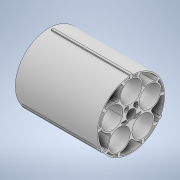
# Autodesk Inventor part: Engine
Saved by Autodesk Inventor 2020 (Build 240168000, 168)
## iProperties
Created: 2022-02-05
Part Number: Engine
Material: Generisch
Document SubType Name: Modeling
Designer: sp
Density: 1 g/cm^3
Appearance: Vorgabe
Author: sp
Autodesk Inventor part; units mm, degrees
ref_plane "YZ Plane" through (0, 0, 0) normal (1, 0, 0) x (0, 1, 0)
ref_plane "XZ Plane" through (0, 0, 0) normal (0, 1, 0) x (-1, 0, 0)
ref_plane "XY Plane" through (0, 0, 0) normal (0, 0, 1) x (1, 0, 0)
sketch "Skizze1" plane through (0, 0, 0) normal (1, 0, 0) x (0, 1, 0)
  circle A0 centre (0, 0) radius 30 construction
  circle A1 centre (17.5, 0) radius 9.5
  circle A2 centre (17.5, 0) radius 10.5
  circle A3 centre (5.4078, 16.6435) radius 9.5
  circle A4 centre (5.4078, 16.6435) radius 10.5
  circle A5 centre (-14.1578, 10.2862) radius 9.5
  circle A6 centre (-14.1578, 10.2862) radius 10.5
  circle A7 centre (-14.1578, -10.2862) radius 9.5
  circle A8 centre (-14.1578, -10.2862) radius 10.5
  circle A9 centre (5.4078, -16.6435) radius 9.5
  circle A10 centre (5.4078, -16.6435) radius 10.5
  circle A11 centre (0, 0) radius 4
  circle A12 centre (0, 0) radius 30
  circle A13 centre (0, 0) radius 29
  dimension "d0" = 60
  dimension "d1" = 17.5
  dimension "d2" = 19
  dimension "d3" = 21
  dimension "d6" = 360
  dimension "d8" = 8
  dimension "d12" = 58
  constraints: 14 centre point, 14 coincident, 1 concentric, 31 other
  measures "d0" diameter of A0
  measures "d1" distance of point (0, 0) point (17.5, 0)
  measures "d2" diameter of A1
  measures "d3" diameter of A2
  measures "d8" diameter of A11
  measures "d12" diameter of A13
extrude "Extrusion1" add sketch "Skizze1" against normal mid plane 70 contours A2 A10 A4 | A4 A2 | A2 A4 A6 | A10 A8 A2 | A2 A10 | A6 A8 A4 | A4 A6 | A10 A8 A6 | A8 A10 | A8 A6
fillet "Rundung1" radius 2 10 edges at (0, 13.1592, -9.5607) (0, -5.0264, -15.4696) (0, -16.2657, 0) (0, -5.0264, 15.4696) (0, 13.1592, 9.5607) (0, 9.7486, -7.0828) (0, 9.7486, 7.0828) (0, -3.7236, 11.4601) (0, -12.0499, 0) (0, -3.7236, -11.4601)
sketch "Skizze2" plane through (35, 0, 0) normal (1, 0, 0) x (0, 0, -1)
  circle A0 centre (0, 0) radius 30
  circle A1 centre (0, 0) radius 29
  dimension "d13" = 60
  dimension "d14" = 58
  constraints: 2 centre point, 2 coincident
  measures "d13" diameter of A0
  measures "d14" diameter of A1
extrude "Extrusion2" add sketch "Skizze2" against normal blind 70
sketch "Skizze3" plane through (0, 0, 0) normal (1, 0, 0) x (0, 1, 0)
  line L0 (35.299, 0) -> (22.394, 0) construction
  line L1 (46.9219, 0) -> (-63.2802, 0) construction
  arc A0 (17.2478, -10.497) -> (17.2478, 10.497) centre (17.5, 0) ccw projected
  line L2 (27.9523, 1) -> (30.9523, 1)
  line L3 (30.9523, 1) -> (30.9523, -1)
  line L4 (30.9523, -1) -> (27.9523, -1)
  line L5 (27.9523, -1) -> (27.9523, 1)
  point P0 (0, 0)
  point P1 (29.9278, 0)
  dimension "d17" = 2
  dimension "d18" = 3
  constraints: 12 end point, 3 horizontal, 3 point on line, 2 parallel, 1 perpendicular, 1 point on circle, 1 other
  measures "d17" distance between parallel lines of L4 L2
  measures "d18" distance between parallel lines of L5 L3
extrude "Extrusion3" add sketch "Skizze3" against normal mid plane 70
pattern_circular "Runde Anordnung1" count 3 over 360 about axis through (-10, 0, 0) along (1, 0, 0) of "Extrusion3"
sketch "Skizze4" plane through (35, 0, 0) normal (1, 0, 0) x (0, 0, -1)
  circle A0 centre (0, 0) radius 4.15
  line L0 (0, 35.2809) -> (0, -56.9195) construction
  line L1 (-52.5037, 0) -> (61.4633, 0) construction
  line L2 (-2.25, 7.6891) -> (2.25, 7.6891)
  line L3 (2.25, 7.6891) -> (2.25, 4.15)
  line L4 (2.25, 4.15) -> (-2.25, 4.15)
  line L5 (-2.25, 4.15) -> (-2.25, 7.6891)
  line L6 (-2.25, 4.15) -> (-2.25, 3.4871)
  line L7 (2.25, 4.15) -> (2.25, 3.4871)
  line L8 (-7.6891, -2.25) -> (-7.6891, 2.25)
  line L9 (-4.15, 2.25) -> (-3.4871, 2.25)
  line L10 (-7.6891, 2.25) -> (-4.15, 2.25)
  line L11 (-4.15, -2.25) -> (-3.4871, -2.25)
  line L12 (-4.15, -2.25) -> (-7.6891, -2.25)
  line L13 (2.25, -7.6891) -> (-2.25, -7.6891)
  line L14 (-2.25, -4.15) -> (-2.25, -3.4871)
  line L15 (-2.25, -7.6891) -> (-2.25, -4.15)
  line L16 (2.25, -4.15) -> (2.25, -3.4871)
  line L17 (2.25, -4.15) -> (2.25, -7.6891)
  line L18 (7.6891, 2.25) -> (7.6891, -2.25)
  line L19 (4.15, -2.25) -> (3.4871, -2.25)
  line L20 (7.6891, -2.25) -> (4.15, -2.25)
  line L21 (4.15, 2.25) -> (3.4871, 2.25)
  line L22 (4.15, 2.25) -> (7.6891, 2.25)
  circle A1 centre (0, 0.0588) radius 5
  point P0 (4.4943, 2.25)
  point P1 (2.25, 4.5239)
  point P2 (-2.25, 4.5239)
  point P3 (-4.4943, 2.25)
  point P4 (-4.435, -2.25)
  point P5 (-2.25, -4.4064)
  point P6 (2.25, -4.4064)
  point P7 (4.435, -2.25)
  dimension "d25" = 8.3
  dimension "d26" = 4.5
  dimension "d29" = 360
  dimension "d31" = 10
  constraints: 46 end point, 3 coincident, 3 parallel, 3 point on line, 2 centre point, 2 horizontal, 2 point on circle, 2 vertical, 1 perpendicular, 48 other
  measures "d25" diameter of A0
  measures "d26" distance of L2.start L2.end
  measures "d31" diameter of A1
extrude "Extrusion4" add sketch "Skizze4" against normal blind 70 contours A0 L21 L22 A1 L20 L19 | A0 L7 L3 A1 L22 L21 | L19 L20 A1 L17 L16 A0 | A0 L4 L7 | L16 L17 A1 L15 L14 A0 | L4 L5 A1 L3 | A0 L6 L4 | L22 L18 L20 A1 | L14 L15 A1 L12 L11 A0 | A0 L9 L10 A1 L5 L6 | A1 L5 L2 L3 | L11 L12 A1 L10 L9 A0 | L17 L13 L15 A1 | A1 L12 L8 L10
sketch "Skizze5" plane through (35, 0, 0) normal (1, 0, 0) x (0, 0, -1)
  line L0 (-7.6891, -2.25) -> (-4.435, -2.25) projected
  arc A0 (-7.6837, 2.25) -> (-7.6891, 2.2346) centre (-16.6435, 5.4078) ccw projected
  line L1 (-7.6891, -2.25) -> (-8.8329, -2.25)
  line L2 (-8.8329, -2.25) -> (-8.8329, 0)
  line L3 (-8.8329, 0) -> (-7.6891, 0)
  line L4 (-7.6891, 0) -> (-7.6891, -2.25)
  line L5 (4.435, -2.25) -> (7.6891, -2.25) projected
  line L6 (7.6891, -2.25) -> (8.9003, -2.25)
  line L7 (8.9003, -2.25) -> (8.9003, 0)
  line L8 (8.9003, 0) -> (7.6891, 0)
  line L9 (7.6891, 0) -> (7.6891, -2.25)
  line L10 (-2.25, -7.3999) -> (-2.25, -4.4064) projected
  circle A1 centre (10.2862, -14.1578) radius 9.5 projected
  line L11 (-2.25, -7.3999) -> (2.2661, -7.3999)
  line L12 (2.2661, -7.3999) -> (2.2661, -9.0659)
  line L13 (2.2661, -9.0659) -> (-2.25, -9.0659)
  line L14 (-2.25, -9.0659) -> (-2.25, -7.3999)
  point P0 (0, 0)
  constraints: 24 end point, 6 parallel, 3 horizontal, 3 perpendicular, 1 point on circle, 1 point on line, 2 other
extrude "Extrusion5" add sketch "Skizze5" against normal blind 70 contours L2 L3 A0 | A0 L3 L4 L1 L2 | L9 L8 L7 L6 | L13 L14 L11 L12
fillet "Rundung3" radius 2 5 edges at (0, -7.3999, -2.25) (0, -7.3999, 2.25) (0, 2.25, 6.6296) (0, 4.5239, -2.25) (0, 2.25, -4.4943)
fillet "Rundung4" radius 2 3 edges at (0, 2.25, 4.4943) (0, 7.2439, -2.25) (0, 2.25, -6.6296)
sketch "Skizze6" plane through (-35, 0, 0) normal (-1, 0, 0) x (0, 0, 1)
  circle A0 centre (0, 0) radius 4.15
  circle A1 centre (0, 17.5) radius 9.5 projected
  circle A2 centre (0, 17.5) radius 9.5
  circle A3 centre (0, 17.5) radius 10.5
  circle A4 centre (-16.6435, 5.4078) radius 9.5
  circle A5 centre (-16.6435, 5.4078) radius 10.5
  circle A6 centre (-10.2862, -14.1578) radius 9.5
  circle A7 centre (-10.2862, -14.1578) radius 10.5
  circle A8 centre (10.2862, -14.1578) radius 9.5
  circle A9 centre (10.2862, -14.1578) radius 10.5
  circle A10 centre (16.6435, 5.4078) radius 9.5
  circle A11 centre (16.6435, 5.4078) radius 10.5
  circle A12 centre (0, 0) radius 30
  dimension "d40" = 360
  constraints: 12 centre point, 8 coincident, 21 other
extrude "Extrusion6" add sketch "Skizze6" along normal blind 3 contours A3 A11 A5 | A5 A3 | A3 A5 A7 | A11 A9 A3 | A3 A11 | A3 A11 A9 A7 A5 | A7 A5 | A5 A7 A9 | A9 A7 | A7 A9 A11 | A9 A11 | A12
sketch "Skizze7" plane through (35, 0, 0) normal (1, 0, 0) x (0, 0, -1)
  line L0 (0, 66.4596) -> (0, -62.7153) construction
  line L1 (-64.2473, 0) -> (96.1757, 0) construction
  arc A0 (10.497, 17.2478) -> (1, 27.9523) centre (0, 17.5) ccw construction
  arc A1 (-1, 27.9523) -> (-10.497, 17.2478) centre (0, 17.5) ccw construction
  line L2 (0, 17.5) -> (11.9823, 34.7083) construction
  line L3 (0, 17.5) -> (-16.2645, 40.8581) construction
  line L4 (4.6539, 26.3161) -> (6.6539, 24.9235)
  line L5 (-6.6571, 24.9281) -> (-4.6571, 26.3208)
  circle A2 centre (0, 17.5) radius 9.5 projected
  circle A3 centre (0, 17.5) radius 9.5 projected
  line L6 (-4.6571, 26.3208) -> (-6.4085, 28.8359)
  line L7 (-6.6571, 24.9281) -> (-8.8554, 28.0851)
  line L8 (4.6539, 26.3161) -> (6.4703, 28.9247)
  line L9 (6.6539, 24.9235) -> (8.883, 28.1247)
  line L10 (8.883, 28.1247) -> (6.4703, 28.9247)
  line L11 (-6.4085, 28.8359) -> (-8.8554, 28.0851)
  point P0 (0, 0)
  point P1 (6, 26.1168)
  point P2 (-6, 26.1168)
  dimension "d44" = 6
  dimension "d45" = 6
  dimension "d46" = 2
  dimension "d47" = 2
  dimension "d48" = 0.3943
  dimension "d49" = 0.4
  dimension "d50" = 90
  dimension "d51" = 90
  dimension "d52" = 90
  dimension "d53" = 90
  constraints: 24 end point, 5 point on line, 2 point on circle, 2 symmetric about line, 1 horizontal, 1 vertical
  measures "d44" distance from line of L0 point (-6, 26.117)
  measures "d45" distance from line of L0 point (6, 26.117)
  measures "d46" horizontal distance of L4.start L4.end
  measures "d47" horizontal distance of L5.start L5.end
  measures "d48" distance edge to line of A2 L4
  measures "d49" distance edge to line of A3 L5
  measures "d50" angle of L4 L9
  measures "d51" angle of L4 L8
  measures "d52" angle of L6 L5
  measures "d53" angle of L5 L7
extrude "Extrusion7" add sketch "Skizze7" against normal blind 70 contours L8 L10 L9 L4 | L7 L11 L6 L5
pattern_circular "Runde Anordnung2" count 5 over 360 about axis through (-10, 0, 0) along (1, 0, 0) of "Extrusion7"
